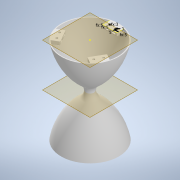
# Autodesk Inventor part: Timglas_main
Saved by Autodesk Inventor 2020.2 (Build 242310000, 310)
## iProperties
Created: 2020-02-13
Part Number: Timglas_main
Material: Generic
Document SubType Name: Modeling
Designer: linus
Density: 1 g/cm^3
Appearance: Default
Author: linus
Autodesk Inventor part; units mm, degrees
ref_plane "YZ Plane" through (0, 0, 0) normal (1, 0, 0) x (0, 1, 0)
ref_plane "XY Plane" through (0, 0, 0) normal (0, 0, 1) x (1, 0, 0)
sketch "Sketch3" plane through (0, 0, 0) normal (0, 0, 1) x (1, 0, 0)
  line L0 (40, 0) -> (5, 55) construction
  arc A0 (40, 0) -> (5, 55) centre (-45.0569, -15.4908) ccw
  line L1 (5, 60) -> (0, 60) construction
  line L2 (0, 0) -> (40, 0)
  line L3 (40, 0) -> (-40, 0)
  line L4 (5, 55) -> (5, 65) construction
  arc A1 (5, 65) -> (40, 120) centre (-45.0569, 135.4908) ccw
  line L5 (0, 120) -> (40, 120)
  line L6 (5, 65) -> (5, 55)
  line L7 (0, 120) -> (0, 0)
  point P0 (5, 55)
  dimension "d40" = 40
  dimension "d49" = 86.456
  dimension "d50" = 80
  dimension "d51" = 120
  dimension "d52" = 55
  dimension "d54" = 10
  dimension "d55" = 5
  dimension "d58" = 5
  dimension "d59" = 5
  constraints: 16 end point, 4 point on circle, 4 symmetric about line, 2 centre point, 1 collinear, 1 point on line, 1 vertical, 1 other
  measures "d40" distance of L2.start L0.start
  measures "d49" radius of A0
  measures "d50" distance of L0.start L3.end
  measures "d51" distance between parallel lines of L5 L2
  measures "d52" vertical distance of L0.start L0.end
  measures "d54" distance of L4.start L4.end
  measures "d55" distance between parallel lines of L7 L4
  measures "d58" distance from line of L7 L1.start
  measures "d59" distance of L1.start L1.end
revolve "Revolution1" add sketch "Sketch3" angle 360 about axis through (0, 120, 0) along (0, -1, 0)
fillet "Fillet1" radius 11.525 2 edges at (-5, 65, 0) (-5, 55, 0)
shell "Shell2" thickness 1.2 removed faces 2 at (6.6991, 120, 6.2575) at (-6.0893, 0, -8.2294)
sketch "Sketch4" plane through (0, 120, 0) normal (0, 1, 0) x (1, 0, 0)
  circle A0 centre (0, 0) radius 38.78 projected
  line L0 (-10, 37.4685) -> (-10, 27.4685)
  line L1 (-10, 27.4685) -> (10, 27.4685)
  line L2 (10, 27.4685) -> (10, 37.4685)
  arc A1 (10, 37.4685) -> (-10, 37.4685) centre (0, 0) ccw
  dimension "d65" = 10
  dimension "d66" = 20
  dimension "d67" = 10
  constraints: 6 end point, 4 point on circle, 2 perpendicular, 1 centre point, 1 concentric, 1 vertical
  measures "d65" distance of L0.start L0.end
  measures "d66" distance of L0.end L1.end
  measures "d67" distance of L1.end L2.end
extrude "Extrusion1" add sketch "Sketch4" against normal blind 5 contours L2 L1 L0 A0 picked at (1.1224, 31.1902)
ref_plane "Work Plane2" through (0, 120, 0) normal (0, 1, 0) x (1, 0, 0)
sketch "Sketch6" plane through (0, 120, 0) normal (0, 1, 0) x (1, 0, 0)
  circle A0 centre (-5, 32.4685) radius 1.5
  circle A1 centre (5, 32.4685) radius 1.5
  line L0 (-10, 27.4685) -> (10, 27.4685) projected
  line L1 (10, 27.4685) -> (10, 37.4685) projected
  line L2 (-10, 37.4685) -> (-10, 27.4685) projected
  point P0 (0, 0)
  dimension "d84" = 3
  dimension "d85" = 3
  dimension "d86" = 5
  dimension "d87" = 5
  dimension "d88" = 5
  dimension "d89" = 5
  constraints: 2 centre point
  measures "d84" diameter of A0
  measures "d85" diameter of A1
  measures "d86" distance from line of L0 A1.centre
  measures "d87" distance from line of L1 A1.centre
  measures "d88" distance from line of L0 A0.centre
  measures "d89" distance from line of L2 A0.centre
extrude "Extrusion3" cut sketch "Sketch6" against normal blind 6
sketch "Sketch7" plane through (-10, 120, -27.4685) normal (0, 0, 1) x (1, 0, 0)
  line L0 (2.25, -1.6) -> (7.75, -1.6)
  line L1 (7.75, -1.6) -> (7.75, -3.4)
  line L2 (7.75, -3.4) -> (2.25, -3.4)
  line L3 (2.25, -3.4) -> (2.25, -1.6)
  line L4 (3.5, -2) -> (6.5, -2) construction
  line L5 (6.5, -2) -> (6.5, -3) construction
  line L6 (6.5, -3) -> (3.5, -3) construction
  line L7 (3.5, -3) -> (3.5, -2) construction
  line L8 (0, 0) -> (0, -5) projected
  line L9 (20, -5) -> (0, -5) projected
  line L10 (17.75, -1.6) -> (12.25, -1.6)
  line L11 (12.25, -1.6) -> (12.25, -3.4)
  line L12 (12.25, -3.4) -> (17.75, -3.4)
  line L13 (17.75, -3.4) -> (17.75, -1.6)
  line L14 (13.5, -2) -> (16.5, -2) construction
  line L15 (16.5, -2) -> (16.5, -3) construction
  line L16 (16.5, -3) -> (13.5, -3) construction
  line L17 (13.5, -3) -> (13.5, -2) construction
  line L18 (20, 0) -> (20, -5) projected
  point P0 (10, -120)
  dimension "d92" = 5.5
  dimension "d93" = 1.8
  dimension "d94" = 3
  dimension "d95" = 1
  dimension "d96" = 1.25
  dimension "d97" = 0.4
  dimension "d99" = 1.6
  dimension "d100" = 3.5
  dimension "d101" = 5.5
  dimension "d102" = 1.8
  dimension "d103" = 3
  dimension "d104" = 1
  dimension "d105" = 1.25
  dimension "d106" = 0.4
  dimension "d107" = 1.6
  dimension "d108" = 3.5
  constraints: 32 end point, 8 parallel, 4 horizontal, 4 perpendicular
  measures "d92" distance of L1.end L2.end
  measures "d93" distance of L0.end L1.end
  measures "d94" distance of L5.end L6.end
  measures "d95" distance of L4.end L5.end
  measures "d96" distance between parallel lines of L3 L7
  measures "d97" distance between parallel lines of L0 L4
  measures "d99" distance between parallel lines of L9 L2
  measures "d100" distance between parallel lines of L8 L7
  measures "d101" distance of L12.end L11.end
  measures "d102" distance of L11.end L10.end
  measures "d103" distance of L15.end L16.end
  measures "d104" distance of L14.end L15.end
  measures "d105" distance between parallel lines of L13 L15
  measures "d106" distance between parallel lines of L10 L14
  measures "d107" distance between parallel lines of L9 L12
  measures "d108" distance between parallel lines of L18 L15
extrude "Extrusion4" cut sketch "Sketch7" against normal blind 7.75
fillet "Fillet2" radius 1 5 edges at (-10, 117.5, -27.4685) (10, 117.5, -27.4685) (-10, 115, -31.909) (10, 115, -31.909) (0, 115, -27.4685)
pattern_circular "Circular Pattern2" count 3 over 360 about axis through (0, -10, 0) along (0, 1, 0) of "Extrusion1", "Extrusion3", "Extrusion4", "Fillet2"
ref_plane "Work Plane3" through (0, 60, 0) normal (0, 1, 0) x (-1, 0, 0)
mirror "Mirror1" about plane through (0, 60, 0) normal (0, 1, 0) of "Extrusion1", "Extrusion3", "Extrusion4", "Fillet2", "Circular Pattern2"
body "Solid1"
